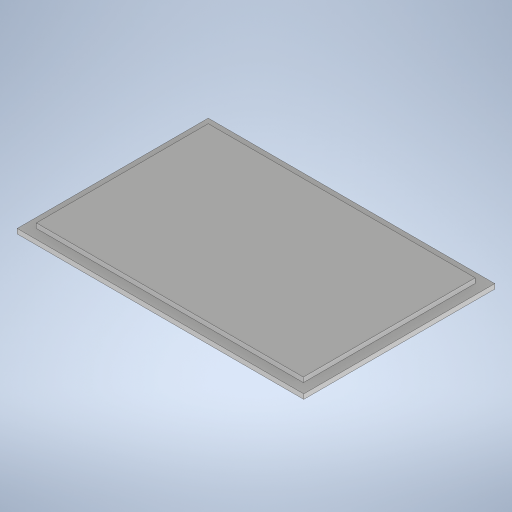
# Autodesk Inventor part: Lid442
Saved by Autodesk Inventor 2024 (Build 280153000, 153)
## iProperties
Created: 2023-11-19
Part Number: Lid442
Material: Generic
Document SubType Name: Modeling
Designer: nickiverson
Density: 1 g/cm^3
Appearance: Default
Author: nickiverson
Autodesk Inventor part; units mm, degrees
ref_plane "YZ Plane" through (0, 0, 0) normal (1, 0, 0) x (0, 1, 0)
ref_plane "XZ Plane" through (0, 0, 0) normal (0, 1, 0) x (-1, 0, 0)
ref_plane "XY Plane" through (0, 0, 0) normal (0, 0, 1) x (1, 0, 0)
sketch "Sketch1" plane through (0, 0, 0) normal (0, 1, 0) x (-1, 0, 0)
  line L0 (0, 0) -> (-152.4, 0)
  line L1 (-152.4, 0) -> (-152.4, -101.6)
  line L2 (-152.4, -101.6) -> (0, -101.6)
  line L3 (0, -101.6) -> (0, 0)
  dimension "d0" = 152.4
  dimension "d1" = 101.6
  constraints: 8 end point, 2 parallel, 1 horizontal, 1 perpendicular
  measures "d0" distance of L2.end L1.end
  measures "d1" distance of L1.end L0.end
extrude "Extrusion1" add sketch "Sketch1" along normal blind 2.54
sketch "Sketch6" plane through (0, 2.54, 0) normal (0, 1, 0) x (1, 0, 0)
  line L0 (0, 0) -> (152.4, 0) projected
  line L1 (152.4, 101.6) -> (0, 101.6) projected
  line L2 (81.7554, 101.6) -> (86.8354, 101.6)
  line L3 (147.1184, 5.08) -> (5.08, 5.08)
  line L4 (5.08, 5.08) -> (5.08, 96.52)
  line L5 (5.08, 96.52) -> (147.1184, 96.52)
  line L6 (147.1184, 96.52) -> (147.1184, 5.08)
  constraints: 10 end point, 2 parallel, 2 point on line, 1 horizontal, 1 perpendicular
extrude "Extrusion6" add sketch "Sketch6" along normal blind 2.54
body "Solid1"
